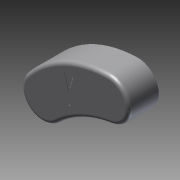
# Autodesk Inventor part: Y Button
Saved by Autodesk Inventor 2012 SP1 (Build 160190100, 190)
## iProperties
Created: 2011-12-08
Part Number: Y Button
Material: Default
Document SubType Name: Modeling
Designer: 133098
Density: 1 g/cm^3
Author: 133098
Autodesk Inventor part; units mm, degrees
ref_plane "YZ Plane" through (0, 0, 0) normal (1, 0, 0) x (0, 1, 0)
ref_plane "XZ Plane" through (0, 0, 0) normal (0, 1, 0) x (-1, 0, 0)
ref_plane "XY Plane" through (0, 0, 0) normal (0, 0, 1) x (1, 0, 0)
sketch "Sketch2" plane through (0, 0, 0) normal (0, 0, 1) x (1, 0, 0)
  arc A0 (28.877, 19.587) -> (33.7764, 14.5025) centre (31.3521, 17.0692) ccw
  arc A1 (43.0166, 18.9913) -> (42.3235, 26.0077) centre (42.4773, 22.4804) ccw
  arc A2 (43.0166, 18.9913) -> (33.7516, 14.4793) centre (45.6813, 1.751) ccw
  arc A3 (42.4773, 26.011) -> (28.3906, 18.9913) centre (42.7991, 7.7213) ccw
  point P0 (0, 0)
  point P1 (43.3585, 19.0616)
  constraints: 14 point on circle, 4 centre point, 1 tangent
extrude "Extrusion2" add sketch "Sketch2" along normal blind 5.08 contours A3 A1 A2 A0
fillet "Fillet5" radius 0.635 6 edges at (42.4004, 26.0095, 5.08) (28.6307, 19.2917, 5.08) (38.0586, 17.4425, 5.08) (33.764, 14.4909, 5.08) (45.9976, 22.7509, 5.08) (29.0787, 14.368, 5.08)
sketch "Sketch3" plane through (0, 0, 5.08) normal (0, 0, 1) x (1, 0, 0)
  line L0 (35.098, 22.767) -> (40.3325, 22.767) construction
  line L1 (40.3325, 22.767) -> (40.3325, 19.1255) construction
  line L2 (40.3325, 19.1255) -> (35.098, 19.1255) construction
  line L3 (35.098, 19.1255) -> (35.098, 22.767) construction
  line L4 (36.881, 22.767) -> (36.1282, 20.2887)
  line L5 (36.1282, 20.2887) -> (36.1282, 18.322)
  line L6 (36.1282, 18.322) -> (35.8328, 18.322)
  line L7 (35.8328, 18.322) -> (35.8328, 20.2275)
  line L8 (35.8328, 20.2275) -> (35.0799, 22.767)
  line L9 (35.0799, 22.767) -> (35.4077, 22.767)
  line L10 (35.4077, 22.767) -> (35.9841, 20.8002)
  line L11 (35.9841, 20.8002) -> (36.5676, 22.767)
  line L12 (36.5676, 22.767) -> (36.881, 22.767)
  point P0 (0, 0)
  constraints: 2 other
extrude "Extrusion3" cut sketch "Sketch3" against normal blind 0.0635
body "Solid2"
